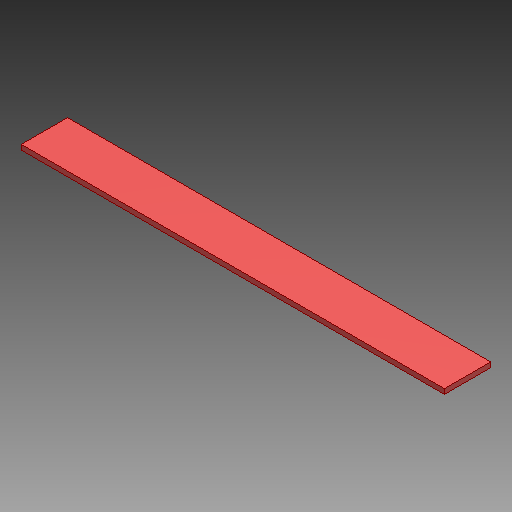
# Autodesk Inventor part: ak
Saved by Autodesk Inventor 2017 (Build 210142000, 142)
## iProperties
Created: 2015-10-11
Part Number: ak
Material: Generic
Document SubType Name: Modeling
Designer: daniel
Density: 1 g/cm^3
Appearance: Default
Author: daniel
Autodesk Inventor part; units mm, degrees
ref_plane "YZ Plane" through (0, 0, 0) normal (1, 0, 0) x (0, 1, 0)
ref_plane "XZ Plane" through (0, 0, 0) normal (0, 1, 0) x (-1, 0, 0)
ref_plane "XY Plane" through (0, 0, 0) normal (0, 0, 1) x (1, 0, 0)
derived "base.ipt"
sketch "sketch_projected_dwg" plane through (0, 0, 0) normal (0, 0, 1) x (1, 0, 0)
  line L0 (2003.2921, -140.5669) -> (2003.2921, -170.5669)
  line L1 (2003.2921, -170.5669) -> (2024.6921, -170.5669)
  line L2 (2024.6921, -170.5669) -> (2024.6921, -140.5669)
  line L3 (2024.6921, -140.5669) -> (2028.9921, -140.5669)
  line L4 (2028.9921, -140.5669) -> (2028.9921, -174.8669)
  line L5 (2028.9921, -174.8669) -> (2048.9921, -174.8669)
  line L6 (2048.9921, -174.8669) -> (2048.9921, -170.5669)
  line L7 (2048.9921, -170.5669) -> (2063.9921, -170.5669)
  line L8 (2063.9921, -170.5669) -> (2063.9921, -110.5669)
  line L9 (2063.9921, -110.5669) -> (2048.9921, -110.5669)
  line L10 (2048.9921, -110.5669) -> (2048.9921, -106.2669)
  line L11 (2048.9921, -106.2669) -> (2028.9921, -106.2669)
  line L12 (2028.9921, -106.2669) -> (2028.9921, -110.5669)
  line L13 (2028.9921, -110.5669) -> (1998.9921, -110.5669)
  line L14 (1998.9921, -110.5669) -> (1998.9921, -106.2669)
  line L15 (1998.9921, -106.2669) -> (1978.9921, -106.2669)
  line L16 (1978.9921, -106.2669) -> (1978.9921, -110.5669)
  line L17 (1978.9921, -110.5669) -> (1963.9921, -110.5669)
  line L18 (1963.9921, -110.5669) -> (1963.9921, -170.5669)
  line L19 (1963.9921, -170.5669) -> (1978.9921, -170.5669)
  line L20 (1978.9921, -170.5669) -> (1978.9921, -174.8669)
  line L21 (1978.9921, -174.8669) -> (1998.9921, -174.8669)
  line L22 (1998.9921, -174.8669) -> (1998.9921, -140.5669)
  line L23 (1998.9921, -140.5669) -> (2003.2921, -140.5669)
  line L24 (2003.2921, -228.8911) -> (2003.2921, -258.8911)
  line L25 (2003.2921, -258.8911) -> (1998.9921, -258.8911)
  line L26 (1998.9921, -258.8911) -> (1998.9921, -228.8911)
  line L27 (1998.9921, -228.8911) -> (1980.0921, -228.8911)
  line L28 (1980.0921, -228.8911) -> (1980.0921, -288.8911)
  line L29 (1980.0921, -288.8911) -> (2047.8921, -288.8911)
  line L30 (2047.8921, -288.8911) -> (2047.8921, -228.8911)
  line L31 (2047.8921, -228.8911) -> (2028.9921, -228.8911)
  line L32 (2028.9921, -228.8911) -> (2028.9921, -258.8911)
  line L33 (2028.9921, -258.8911) -> (2024.6921, -258.8911)
  line L34 (2024.6921, -258.8911) -> (2024.6921, -228.8911)
  line L35 (2024.6921, -228.8911) -> (2003.2921, -228.8911)
  circle A0 centre (2043.9921, -271.0911) radius 6
  circle A1 centre (2013.9921, -271.0911) radius 4.7571
  circle A2 centre (1983.9921, -271.0911) radius 6
  line L36 (2369.6683, 1.7867) -> (2369.6683, -98.2133)
  line L37 (2463.2683, 1.7867) -> (2463.2683, -98.2133)
  line L38 (2382.5683, -263.5692) -> (2382.5683, -363.5692)
  line L39 (2450.3683, -263.5692) -> (2450.3683, -363.5692)
  line L40 (2322.5683, -263.5692) -> (2382.5683, -263.5692)
  line L41 (2382.5683, -263.5692) -> (2416.4683, -263.5692)
  line L42 (2416.4683, -263.5692) -> (2450.3683, -263.5692)
  line L43 (2450.3683, -263.5692) -> (2510.3683, -263.5692)
  line L44 (2510.3683, -263.5692) -> (2510.3683, -333.5692)
  line L45 (2510.3683, -333.5692) -> (2480.3683, -363.5692)
  line L46 (2480.3683, -363.5692) -> (2352.5683, -363.5692)
  line L47 (2352.5683, -363.5692) -> (2322.5683, -333.5692)
  line L48 (2322.5683, -333.5692) -> (2322.5683, -263.5692)
  line L49 (2401.4683, -278.5692) -> (2405.7683, -278.5692)
  line L50 (2405.7683, -278.5692) -> (2405.7683, -298.5692)
  line L51 (2405.7683, -298.5692) -> (2401.4683, -298.5692)
  line L52 (2401.4683, -298.5692) -> (2401.4683, -278.5692)
  line L53 (2427.1683, -278.5692) -> (2431.4683, -278.5692)
  line L54 (2431.4683, -278.5692) -> (2431.4683, -298.5692)
  line L55 (2431.4683, -298.5692) -> (2427.1683, -298.5692)
  line L56 (2427.1683, -298.5692) -> (2427.1683, -278.5692)
  line L57 (2427.1683, -328.5692) -> (2431.4683, -328.5692)
  line L58 (2431.4683, -328.5692) -> (2431.4683, -348.5692)
  line L59 (2431.4683, -348.5692) -> (2427.1683, -348.5692)
  line L60 (2427.1683, -348.5692) -> (2427.1683, -328.5692)
  line L61 (2401.4683, -328.5692) -> (2405.7683, -328.5692)
  line L62 (2405.7683, -328.5692) -> (2405.7683, -348.5692)
  line L63 (2405.7683, -348.5692) -> (2401.4683, -348.5692)
  line L64 (2401.4683, -348.5692) -> (2401.4683, -328.5692)
  line L65 (2401.4683, -63.2133) -> (2405.7683, -63.2133)
  line L66 (2405.7683, -63.2133) -> (2405.7683, -83.2133)
  line L67 (2405.7683, -83.2133) -> (2401.4683, -83.2133)
  line L68 (2401.4683, -83.2133) -> (2401.4683, -63.2133)
  line L69 (2373.9683, -63.2133) -> (2378.2683, -63.2133)
  line L70 (2378.2683, -63.2133) -> (2378.2683, -83.2133)
  line L71 (2378.2683, -83.2133) -> (2373.9683, -83.2133)
  line L72 (2373.9683, -83.2133) -> (2373.9683, -63.2133)
  line L73 (2373.9683, -13.2133) -> (2378.2683, -13.2133)
  line L74 (2378.2683, -13.2133) -> (2378.2683, -33.2133)
  line L75 (2378.2683, -33.2133) -> (2373.9683, -33.2133)
  line L76 (2373.9683, -33.2133) -> (2373.9683, -13.2133)
  line L77 (2401.4683, -13.2133) -> (2405.7683, -13.2133)
  line L78 (2405.7683, -13.2133) -> (2405.7683, -33.2133)
  line L79 (2405.7683, -33.2133) -> (2401.4683, -33.2133)
  line L80 (2401.4683, -33.2133) -> (2401.4683, -13.2133)
  line L81 (2427.1683, -13.2133) -> (2431.4683, -13.2133)
  line L82 (2431.4683, -13.2133) -> (2431.4683, -33.2133)
  line L83 (2431.4683, -33.2133) -> (2427.1683, -33.2133)
  line L84 (2427.1683, -33.2133) -> (2427.1683, -13.2133)
  line L85 (2454.6683, -13.2133) -> (2458.9683, -13.2133)
  line L86 (2458.9683, -13.2133) -> (2458.9683, -33.2133)
  line L87 (2458.9683, -33.2133) -> (2454.6683, -33.2133)
  line L88 (2454.6683, -33.2133) -> (2454.6683, -13.2133)
  line L89 (2454.6683, -63.2133) -> (2458.9683, -63.2133)
  line L90 (2458.9683, -63.2133) -> (2458.9683, -83.2133)
  line L91 (2458.9683, -83.2133) -> (2454.6683, -83.2133)
  line L92 (2454.6683, -83.2133) -> (2454.6683, -63.2133)
  line L93 (2427.1683, -63.2133) -> (2431.4683, -63.2133)
  line L94 (2431.4683, -63.2133) -> (2431.4683, -83.2133)
  line L95 (2431.4683, -83.2133) -> (2427.1683, -83.2133)
  line L96 (2427.1683, -83.2133) -> (2427.1683, -63.2133)
  line L97 (2508.9683, -98.2133) -> (2458.9683, -98.2133)
  line L98 (2458.9683, 61.7867) -> (2508.9683, 61.7867)
  line L99 (2508.9683, 61.7867) -> (2508.9683, 1.7867)
  line L100 (2508.9683, 1.7867) -> (2587.5683, 1.7867)
  line L101 (2587.5683, 1.7867) -> (2587.5683, -13.2133)
  line L102 (2587.5683, -13.2133) -> (2591.8683, -13.2133)
  line L103 (2591.8683, -13.2133) -> (2591.8683, -33.2133)
  line L104 (2591.8683, -33.2133) -> (2587.5683, -33.2133)
  line L105 (2587.5683, -33.2133) -> (2587.5683, -48.2133)
  line L106 (2587.5683, -48.2133) -> (2587.5683, -63.2133)
  line L107 (2587.5683, -63.2133) -> (2591.8683, -63.2133)
  line L108 (2591.8683, -63.2133) -> (2591.8683, -83.2133)
  line L109 (2591.8683, -83.2133) -> (2587.5683, -83.2133)
  line L110 (2587.5683, -83.2133) -> (2587.5683, -98.2133)
  line L111 (2587.5683, -98.2133) -> (2508.9683, -98.2133)
  line L112 (2508.9683, -98.2133) -> (2508.9683, -158.2133)
  line L113 (2508.9683, -158.2133) -> (2397.2842, -158.2133)
  line L114 (2523.2683, 1.7867) -> (2523.2683, -98.2133)
  line L115 (2527.5683, 1.7867) -> (2527.5683, -98.2133)
  line L116 (2373.9683, -158.2133) -> (2373.9683, -98.2133)
  line L117 (2373.9683, -98.2133) -> (2458.9683, -98.2133)
  line L118 (2458.9683, -98.2133) -> (2458.9683, -158.2133)
  circle A3 centre (2446.4683, -116.0133) radius 6
  circle A4 centre (2424.7172, -111.2508) radius 1.5
  circle A5 centre (2416.4683, -116.0133) radius 6.35
  circle A6 centre (2408.2194, -111.2508) radius 1.5
  circle A7 centre (2416.4683, -125.5383) radius 1.5
  circle A8 centre (2386.4683, -116.0133) radius 6
  line L119 (2373.9683, -158.2133) -> (2416.4683, -158.2133)
  line L120 (2416.4683, -158.2133) -> (2458.9683, -158.2133)
  line L121 (2397.2842, -158.2133) -> (2323.9683, -158.2133)
  line L122 (2323.9683, -158.2133) -> (2323.9683, -98.2133)
  line L123 (2323.9683, -98.2133) -> (2245.3683, -98.2133)
  line L124 (2245.3683, -98.2133) -> (2245.3683, -83.2133)
  line L125 (2245.3683, -83.2133) -> (2241.0683, -83.2133)
  line L126 (2241.0683, -83.2133) -> (2241.0683, -63.2133)
  line L127 (2241.0683, -63.2133) -> (2245.3683, -63.2133)
  line L128 (2245.3683, -63.2133) -> (2245.3683, -48.2133)
  line L129 (2245.3683, -48.2133) -> (2245.3683, -33.2133)
  line L130 (2245.3683, -33.2133) -> (2241.0683, -33.2133)
  line L131 (2241.0683, -33.2133) -> (2241.0683, -13.2133)
  line L132 (2241.0683, -13.2133) -> (2245.3683, -13.2133)
  line L133 (2245.3683, -13.2133) -> (2245.3683, 1.7867)
  line L134 (2245.3683, 1.7867) -> (2323.9683, 1.7867)
  line L135 (2323.9683, 1.7867) -> (2323.9683, 61.7867)
  line L136 (2323.9683, -98.2133) -> (2373.9683, -98.2133)
  line L137 (2309.6683, 1.7867) -> (2309.6683, -98.2133)
  line L138 (2305.3683, 1.7867) -> (2305.3683, -98.2133)
  line L139 (2323.9683, 61.7867) -> (2373.9683, 61.7867)
  line L140 (2373.9683, 61.7867) -> (2416.4683, 61.7867)
  line L141 (2416.4683, 61.7867) -> (2458.9683, 61.7867)
  line L142 (2373.9683, 61.7867) -> (2373.9683, 1.7867)
  line L143 (2373.9683, 1.7867) -> (2458.9683, 1.7867)
  line L144 (2458.9683, 1.7867) -> (2458.9683, 61.7867)
  circle A9 centre (2386.4683, 19.5867) radius 6
  circle A10 centre (2416.4683, 19.5867) radius 4.5
  circle A11 centre (2446.4683, 19.5867) radius 6
  line L145 (2508.9683, 1.7867) -> (2458.9683, 1.7867)
  line L146 (2323.9683, 1.7867) -> (2373.9683, 1.7867)
  line L147 (1479.0412, 298.6353) -> (1296.2412, 298.6353)
  line L148 (1296.2412, 298.6353) -> (1296.2412, 233.6353)
  line L149 (1296.2412, 233.6353) -> (1479.0412, 233.6353)
  line L150 (1479.0412, 233.6353) -> (1591.8412, 233.6353)
  line L151 (1591.8412, 233.6353) -> (1774.6412, 233.6353)
  line L152 (1774.6412, 233.6353) -> (1774.6412, 298.6353)
  line L153 (1774.6412, 298.6353) -> (1591.8412, 298.6353)
  line L154 (1591.8412, 298.6353) -> (1479.0412, 298.6353)
  line L155 (1591.8412, 298.6353) -> (1591.8412, 233.6353)
  circle A12 centre (1565.4412, 268.6353) radius 5
  circle A13 centre (1550.9412, 284.1353) radius 1.5
  circle A14 centre (1550.9412, 253.1353) radius 1.5
  circle A15 centre (1535.4412, 268.6353) radius 4.5
  circle A16 centre (1505.4412, 268.6353) radius 5
  circle A17 centre (1519.9412, 253.1353) radius 1.5
  circle A18 centre (1519.9412, 284.1353) radius 1.5
  line L156 (1479.0412, 298.6353) -> (1479.0412, 233.6353)
  line L157 (1479.0412, 177.6353) -> (1479.0412, 112.6353)
  line L158 (1479.0412, 177.6353) -> (1296.2412, 177.6353)
  line L159 (1296.2412, 177.6353) -> (1296.2412, 112.6353)
  line L160 (1296.2412, 112.6353) -> (1774.6412, 112.6353)
  line L161 (1774.6412, 112.6353) -> (1774.6412, 177.6353)
  line L162 (1774.6412, 177.6353) -> (1591.8412, 177.6353)
  line L163 (1591.8412, 177.6353) -> (1479.0412, 177.6353)
  line L164 (1591.8412, 177.6353) -> (1591.8412, 112.6353)
  circle A19 centre (1565.4412, 147.6353) radius 5
  circle A20 centre (1535.4412, 147.6353) radius 4.5
  circle A21 centre (1505.4412, 147.6353) radius 5
  line L165 (1560.4412, 18.4276) -> (1510.4412, 18.4276)
  line L166 (1510.4412, 18.4276) -> (1510.4412, 9.8276)
  line L167 (1510.4412, 9.8276) -> (1510.4412, -6.5724)
  line L168 (1510.4412, -6.5724) -> (1560.4412, -6.5724)
  line L169 (1560.4412, -6.5724) -> (1560.4412, 9.8276)
  line L170 (1560.4412, 9.8276) -> (1560.4412, 18.4276)
  line L171 (1479.0412, 14.1276) -> (1510.4412, 14.1276)
  line L172 (1454.0412, 79.1276) -> (1454.0412, 14.1276)
  line L173 (1454.0412, 14.1276) -> (1479.0412, 14.1276)
  line L174 (1479.0412, 79.1276) -> (1479.0412, 14.1276)
  line L175 (1454.0412, 79.1276) -> (1479.0412, 79.1276)
  line L176 (1479.0412, 79.1276) -> (1591.8412, 79.1276)
  circle A22 centre (1505.4412, 49.1276) radius 5
  circle A23 centre (1535.4412, 49.1276) radius 4.5
  circle A24 centre (1565.4412, 49.1276) radius 5
  line L177 (1591.8412, 79.1276) -> (1591.8412, 14.1276)
  line L178 (1591.8412, 14.1276) -> (1560.4412, 14.1276)
  line L179 (1591.8412, 14.1276) -> (1616.8412, 14.1276)
  line L180 (1616.8412, 79.1276) -> (1616.8412, 14.1276)
  line L181 (1591.8412, 79.1276) -> (1616.8412, 79.1276)
  line L182 (1479.0412, -262.9517) -> (1591.8412, -262.9517)
  line L183 (1479.0412, -262.9517) -> (1479.0412, -327.9517)
  circle A25 centre (1519.9412, -277.4517) radius 1.5
  line L184 (1591.8412, -262.9517) -> (1591.8412, -327.9517)
  circle A26 centre (1565.4412, -292.9517) radius 5
  circle A27 centre (1550.9412, -277.4517) radius 1.5
  circle A28 centre (1550.9412, -308.4517) radius 1.5
  circle A29 centre (1519.9412, -308.4517) radius 1.5
  circle A30 centre (1535.4412, -292.9517) radius 11
  circle A31 centre (1505.4412, -292.9517) radius 5
  line L185 (1479.0412, -327.9517) -> (1510.4412, -327.9517)
  line L186 (1510.4412, -323.6517) -> (1510.4412, -332.2517)
  line L187 (1510.4412, -332.2517) -> (1510.4412, -348.6517)
  line L188 (1510.4412, -348.6517) -> (1560.4412, -348.6517)
  line L189 (1560.4412, -348.6517) -> (1560.4412, -332.2517)
  line L190 (1560.4412, -332.2517) -> (1560.4412, -323.6517)
  line L191 (1560.4412, -323.6517) -> (1510.4412, -323.6517)
  line L192 (1591.8412, -327.9517) -> (1560.4412, -327.9517)
  line L193 (616.2683, 257.5909) -> (616.2683, 503.2909)
  line L194 (616.2683, 503.2909) -> (551.2683, 503.2909)
  line L195 (551.2683, 503.2909) -> (551.2683, 335.4909)
  line L196 (551.2683, 335.4909) -> (546.9683, 335.4909)
  line L197 (546.9683, 335.4909) -> (546.9683, 420.4909)
  line L198 (546.9683, 420.4909) -> (496.9683, 420.4909)
  line L199 (496.9683, 420.4909) -> (496.9683, 335.4909)
  line L200 (496.9683, 335.4909) -> (488.3683, 335.4909)
  line L201 (488.3683, 335.4909) -> (488.3683, 440.4909)
  line L202 (488.3683, 440.4909) -> (122.7683, 440.4909)
  line L203 (122.7683, 440.4909) -> (122.7683, 335.4909)
  line L204 (122.7683, 335.4909) -> (114.1683, 335.4909)
  line L205 (114.1683, 335.4909) -> (114.1683, 420.4909)
  line L206 (114.1683, 420.4909) -> (64.1683, 420.4909)
  line L207 (64.1683, 420.4909) -> (64.1683, 335.4909)
  line L208 (64.1683, 335.4909) -> (59.8683, 335.4909)
  line L209 (59.8683, 335.4909) -> (59.8683, 503.2909)
  line L210 (59.8683, 503.2909) -> (-5.1317, 503.2909)
  line L211 (-5.1317, 503.2909) -> (-5.1317, 257.5909)
  line L212 (496.9683, 400.4909) -> (546.9683, 400.4909)
  line L213 (496.9683, 396.1909) -> (546.9683, 396.1909)
  line L214 (122.7683, 396.1909) -> (488.3683, 396.1909)
  line L215 (488.3683, 400.4909) -> (122.7683, 400.4909)
  line L216 (546.9683, 335.4909) -> (496.9683, 335.4909)
  line L217 (488.3683, 335.4909) -> (122.7683, 335.4909)
  line L218 (551.2683, 326.8909) -> (59.8683, 326.8909)
  line L219 (551.2683, 335.4909) -> (551.2683, 326.8909)
  line L220 (551.2683, 326.8909) -> (551.2683, 261.8909)
  line L221 (616.2683, 257.5909) -> (551.2683, 257.5909)
  line L222 (551.2683, 136.1909) -> (551.2683, 257.5909)
  line L223 (59.8683, 261.8909) -> (551.2683, 261.8909)
  line L224 (551.2683, 257.5909) -> (551.2683, 261.8909)
  line L225 (616.2683, 257.5909) -> (616.2683, 136.1909)
  circle A32 centre (586.2683, 226.8909) radius 5
  circle A33 centre (586.2683, 166.8909) radius 5
  line L226 (616.2683, 136.1909) -> (551.2683, 136.1909)
  line L227 (59.8683, 131.8909) -> (551.2683, 131.8909)
  line L228 (551.2683, 136.1909) -> (551.2683, 131.8909)
  line L229 (59.8683, 257.5909) -> (59.8683, 136.1909)
  line L230 (59.8683, 136.1909) -> (-5.1317, 136.1909)
  line L231 (59.8683, 136.1909) -> (59.8683, 131.8909)
  line L232 (59.8683, 257.5909) -> (59.8683, 261.8909)
  line L233 (-5.1317, 257.5909) -> (59.8683, 257.5909)
  line L234 (-5.1317, 257.5909) -> (-5.1317, 136.1909)
  circle A34 centre (24.8683, 226.8909) radius 5
  circle A35 centre (24.8683, 166.8909) radius 5
  line L235 (59.8683, 335.4909) -> (59.8683, 318.2909)
  line L236 (59.8683, 318.2909) -> (59.8683, 261.8909)
  line L237 (64.1683, 335.4909) -> (114.1683, 335.4909)
  line L238 (114.1683, 396.1909) -> (64.1683, 396.1909)
  line L239 (114.1683, 400.4909) -> (64.1683, 400.4909)
  line L240 (122.7683, 206.8909) -> (488.3683, 206.8909)
  line L241 (122.7683, 206.8909) -> (122.7683, 186.8909)
  line L242 (122.7683, 186.8909) -> (488.3683, 186.8909)
  line L243 (488.3683, 196.8909) -> (488.3683, 186.8909)
  line L244 (488.3683, 206.8909) -> (488.3683, 196.8909)
  line L245 (59.3683, -191.4724) -> (459.3683, -191.4724) construction
  line L246 (1487.6412, -271.5517) -> (1507.6412, -271.5517)
  line L247 (1507.6412, -271.5517) -> (1507.6412, -278.0517)
  line L248 (1507.6412, -278.0517) -> (1487.6412, -278.0517)
  line L249 (1487.6412, -278.0517) -> (1487.6412, -271.5517)
  line L250 (1487.6412, 290.0353) -> (1507.6412, 290.0353)
  line L251 (1507.6412, 290.0353) -> (1507.6412, 283.5353)
  line L252 (1507.6412, 283.5353) -> (1487.6412, 283.5353)
  line L253 (1487.6412, 283.5353) -> (1487.6412, 290.0353)
  line L254 (1563.2412, 169.0353) -> (1583.2412, 169.0353)
  line L255 (1583.2412, 169.0353) -> (1583.2412, 162.5353)
  line L256 (1583.2412, 162.5353) -> (1563.2412, 162.5353)
  line L257 (1563.2412, 162.5353) -> (1563.2412, 169.0353)
  line L258 (1487.6412, 70.5276) -> (1507.6412, 70.5276)
  line L259 (1507.6412, 70.5276) -> (1507.6412, 64.0276)
  line L260 (1507.6412, 64.0276) -> (1487.6412, 64.0276)
  line L261 (1487.6412, 64.0276) -> (1487.6412, 70.5276)
  point P0 (0, 0)
extrude "Extrusion1" add sketch "sketch_projected_dwg" along normal blind 4.3 contours L215 L203 L202 L201
equation "\"d1\" = material_thickness"
equation "\"material_thickness\" = 4.3"
body "Solid1"
